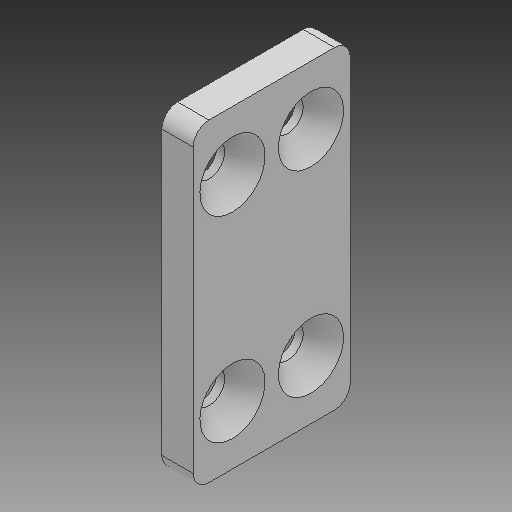
# Autodesk Inventor part: Counter_Support_Ceramic_Leg
Saved by Autodesk Inventor 2017 (Build 210142000, 142)
## iProperties
Created: 2020-01-10
Part Number: Counter_Support_Ceramic_Leg
Material: Generic
Document SubType Name: Modeling
Designer: Christian
Density: 1 g/cm^3
Appearance: Default
Author: Christian
Autodesk Inventor part; units mm, degrees
ref_plane "YZ Plane" through (0, 0, 0) normal (1, 0, 0) x (0, 1, 0)
ref_plane "XZ Plane" through (0, 0, 0) normal (0, 1, 0) x (-1, 0, 0)
ref_plane "XY Plane" through (0, 0, 0) normal (0, 0, 1) x (1, 0, 0)
sketch "Leg_Base_Skt" plane through (0, 0, 0) normal (1, 0, 0) x (0, 1, 0)
  line L0 (-10, -20) -> (10, -20)
  line L1 (10, -20) -> (10, 20)
  line L2 (10, 20) -> (-10, 20)
  line L3 (-10, 20) -> (-10, -20)
  line L4 (-10, -20) -> (10, 20) construction
  line L5 (10, -20) -> (-10, 20) construction
  point P0 (0, 0)
  dimension "d0" = 20
  dimension "d1" = 40
  constraints: 12 end point, 2 midpoint, 2 parallel, 1 horizontal, 1 perpendicular
  measures "d0" distance of L1.end L2.end
  measures "d1" distance of L0.end L1.end
extrude "Leg_Base" add sketch "Leg_Base_Skt" along normal blind 4
sketch "Hole_Base_Skt" plane through (4, 0, 0) normal (1, 0, 0) x (0, 0, -1)
  line L0 (-5, -10) -> (-5, 10) construction
  line L1 (20, 10) -> (-20, 10) projected
  line L2 (-12.5, 0) -> (-12.5, 10) construction
  line L3 (-12.5, 0) -> (-12.5, -10) construction
  line L4 (-20, -10) -> (20, -10) construction
  line L5 (5, -10) -> (5, 10) construction
  line L6 (20, -10) -> (20, 10) construction
  line L7 (5, 0) -> (20, 0) construction
  line L8 (12.5, 0) -> (12.5, 10) construction
  line L9 (12.5, 0) -> (12.5, -10) construction
  line L10 (-20, 10) -> (-20, -10) projected
  line L11 (-20, 0) -> (-5, 0) construction
  point P0 (0, 0)
  point P1 (-12.5, -5)
  point P2 (-12.5, 5)
  point P3 (12.5, -5)
  point P4 (12.5, 5)
  dimension "d7" = 15
  dimension "d8" = 15
  constraints: 16 end point, 10 midpoint, 10 point on line, 3 perpendicular, 1 vertical
  measures "d7" distance between parallel lines of L6 L5
  measures "d8" distance between parallel lines of L10 L0
hole "Hole_Base" at (4, -5, 12.5) at (4, 5, 12.5) at (4, -5, -12.5) at (4, 5, -12.5) direction (-1, 0, 0) diameter 4 end through all countersink diameter 8.3 countersink angle 71.667
fillet "Fillet" radius 2 4 edges at (2, -10, 20) (2, 10, 20) (2, -10, -20) (2, 10, -20)
equation "\"d0\" = block_width"
equation "\"d1\" = ceramic_width + block_height + wood_width"
equation "\"d2\" = screw_head_height + screw_tolerance"
equation "\"d7\" = wood_width"
equation "\"d8\" = block_height"
equation "\"d28\" = screw_body_diam + screw_tolerance"
equation "\"d32\" = screw_head_m"
equation "\"d30\" = screw_head_diam"
equation "\"d33\" = screw_length"
equation "\"d4\" = fillet"
equation "\"tube_diam\" = 31.8"
equation "\"tube_tolerance\" = 0.25"
equation "\"tube_base_height\" = 2"
equation "\"tube_wall_width\" = 3"
equation "\"tube_wall_height\" = 15"
equation "\"screw_wall_width\" = 2"
equation "\"screw_length\" = 12.7"
equation "\"screw_tolerance\" = 1"
equation "\"screw_body_diam\" = 3"
equation "\"screw_head_diam\" = 8.3"
equation "\"screw_head_height\" = 3"
equation "\"screw_spacing\" = 8"
equation "\"block_width\" = 20"
equation "\"block_height\" = 15"
equation "\"ceramic_width\" = 10"
equation "\"wood_width\" = 15"
equation "\"fillet\" = 2"
equation "\"screw_head_m\" = 71.6667deg"
body "Solid1"
